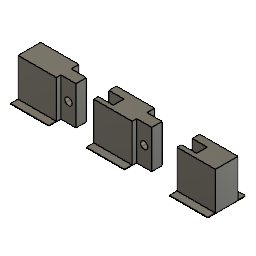
1 inch Epoxy Damn v1 (Autodesk Fusion 360 design; units mm, degrees)
Autodesk Fusion 360 part; units mm, degrees
note: some values were not read from the file. Set by a fixed rule: which sketch regions a step uses.
sketch "Sketch1" plane through (0, 0, 0) normal (1, 0, 0) x (0, 0, -1)
  line L0 (0, 0) -> (2, 0)
  line L1 (2, 0) -> (2, 25)
  line L2 (2, 25) -> (0, 25)
  line L3 (0, 25) -> (0, 0)
  line L4 (2, 25) -> (9, 25)
  line L5 (9, 25) -> (9, 0)
  line L6 (9, 0) -> (2, 0)
  line L7 (2, 0) -> (2, 25)
  line L8 (9, 0) -> (14, 0)
  line L9 (14, 0) -> (14, 25)
  line L10 (14, 25) -> (9, 25)
  line L11 (9, 25) -> (9, 0)
  line L12 (14, 0) -> (19, 0)
  line L13 (19, 0) -> (19, -0.4)
  line L14 (19, -0.4) -> (14, -0.4)
  line L15 (14, -0.4) -> (14, 0)
  line L16 (0, 0) -> (-5, 0)
  line L17 (-5, 0) -> (19, 0)
  line L18 (19, 0) -> (19, -0.4)
  line L19 (19, -0.4) -> (-5, -0.4)
  line L20 (-5, -0.4) -> (-5, 0)
  dimension "d1" = 2
  dimension "d2" = 25
  dimension "d3" = 7
  dimension "d4" = 25
  dimension "d5" = 5
  dimension "d6" = 5
  dimension "d7" = 0.4
  dimension "d8" = 5
  constraint horizontal L0
  constraint vertical L1
  constraint horizontal L2
  constraint vertical L3
  constraint coincident L0.start L3.end
  constraint horizontal L4
  constraint vertical L5
  constraint horizontal L6
  constraint vertical L7
  constraint horizontal L8
  constraint vertical L9
  constraint horizontal L10
  constraint vertical L11
  constraint horizontal L12
  constraint vertical L13
  constraint horizontal L14
  constraint vertical L15
  constraint perpendicular L3 L16
  constraint horizontal L17
  constraint vertical L18
  constraint horizontal L19
  constraint vertical L20
  measures "d1" distance of L0.start L0.end
  measures "d2" distance of L0.start L2.end
  measures "d3" distance of L1.end L4.end
  measures "d4" distance of L1.end L0.end
  measures "d5" distance of L5.end L8.end
  measures "d6" distance of L8.end L12.end
  measures "d7" distance of L8.end L14.end
  measures "d8" distance of L0.start L16.end
extrude "Extrude1" add sketch "Sketch1" along normal blind 25.4 makes body 1
extrude "Extrude2" cut sketch "Sketch1" along normal blind 10 contours L1 L4 L5 L6 L7 L11 L17 bodies 1
extrude "Extrude3" cut 1 faces at (3.3333, 0, -6.6667) along direction (0, -1, 0) blind 0.4 on bodies 1 bodies 1
extrude "Extrude4" add sketch "Sketch1" along normal blind 35.4 and the other way blind -25.4 contours L1 L4 L5 L6 L7 L11 L17 bodies 1
extrude "Extrude5" add 1 faces at (28.7333, 0, -6.6667) along direction (0, -1, 0) blind 0.4 on bodies 1 bodies 1
sketch "Sketch2" plane through (0, 0, -14) normal (0, 0, -1) x (-1, 0, 0)
  line L0 (0, 0) -> (0, 25)
  line L1 (0, 25) -> (-25.4, 25)
  line L2 (-25.4, 25) -> (-25.4, 0)
  line L3 (-25.4, 0) -> (0, 0)
  line L4 (0, 12.5) -> (-10, 12.5)
  circle A0 centre (-5, 12.5) radius 2.4
  dimension "d21" = 10
  dimension "d22" = 4.8
  constraint midpoint L0 L4.start
  constraint perpendicular L0 L4
  constraint midpoint L4 A0.centre
  measures "d21" distance of L4.start L4.end
  measures "d22" diameter of A0
extrude "Extrude6" cut sketch "Sketch2" against normal blind 13.6 contours L4 A0 | L4 A0 bodies 1
extrude "Extrude7" add 1 faces at (8.4667, 16.6667, 0) along direction (0, 0, 1) blind 1 on bodies 1 bodies 1
extrude "Extrude8" add 1 faces at (8.4667, -0.2667, 5) along direction (0, 0, 1) blind 1 on bodies 1 bodies 1
sketch "Sketch3" plane through (0, 0, -14) normal (0, 0, -1) x (-1, 0, 0)
  circle A0 centre (-5, 12.5) radius 2.4
  line L0 (0, 0) -> (0, 25)
  line L1 (0, 25) -> (-25.4, 25)
  line L2 (-25.4, 25) -> (-25.4, 0)
  line L3 (-25.4, 0) -> (0, 0)
  circle A1 centre (-5, 12.5) radius 4.35
  dimension "d29" = 8.7
  constraint concentric A0 A1
  measures "d29" diameter of A1
extrude "Extrude9" cut sketch "Sketch3" against normal blind 4.35 contours A1 bodies 1
chamfer "Chamfer1" distance 1.95 angle 45 1 edges at (9.0556, 14.073, -9.65) on bodies 1
sketch "Sketch4" plane through (0, 0, -9) normal (0, 0, -1) x (-1, 0, 0)
  line L0 (-25.4, -0.4) -> (-25.4, 25)
  line L1 (-25.4, 25) -> (-35.4, 25)
  line L2 (-35.4, 25) -> (-35.4, -0.4)
  line L3 (-35.4, -0.4) -> (-25.4, -0.4)
  line L4 (-35.4, 12.3) -> (-25.4, 12.3)
  circle A0 centre (-30.4, 12.3) radius 2.4
  dimension "d33" = 4.8
  constraint midpoint L2 L4.start
  constraint midpoint L0 L4.end
  constraint midpoint L4 A0.centre
  measures "d33" diameter of A0
extrude "Extrude10" cut sketch "Sketch4" against normal blind 7 contours L4 A0 | L4 A0 bodies 1
copy_body "CopyPasteBodies1" bodies 1 makes body 2
move_body "Move1" bodies 2 to x (1, 0, 0) y (0, 1, 0) z (0, 0, 1) at (-50, 0, 0)
extrude "Extrude11" add 1 faces at (-40, 8.0667, -4.3333) along direction (-1, 0, 0) blind 10 on bodies 2 bodies 2
sketch "Sketch5" plane through (0, 0, -14) normal (0, 0, -1) x (-1, 0, 0)
  circle A0 centre (45, 12.5) radius 4.35
  line L0 (50, 0) -> (50, 25)
  line L1 (50, 25) -> (24.6, 25)
  line L2 (24.6, 25) -> (24.6, 0)
  line L3 (24.6, 0) -> (50, 0)
extrude "Extrude12" add sketch "Sketch5" against normal blind 15 contours A0 bodies 2
copy_body "CopyPasteBodies2" bodies 1 makes body 3
move_body "Move2" bodies 3 to x (1, 0, 0) y (0, 1, 0) z (0, 0, 1) at (55, 0, 0)
extrude "Extrude13" cut 1 faces at (90.4, 16.5333, -6.6667) along direction (-1, 0, 0) blind 10 on bodies 3 bodies 3
move_face "MoveFace1" by (0, 0, 0.1) 2 faces at (30.4598, 3.0356, -9) (-19.5402, 3.0356, -9) on bodies 1 2
equation "d15 = 25.4 mm + 10 mm"
named bodies: "1 inch Damn Middle", "1 inch Damn Back", "1 Inch Damn Front"
